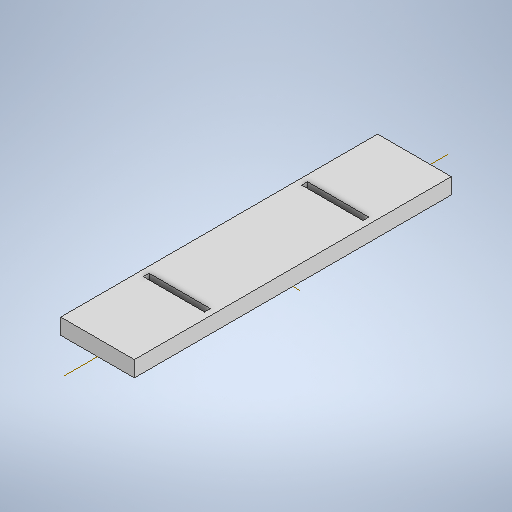
# Autodesk Inventor part: end_wall
Saved by Autodesk Inventor 2025 (Build 290162000, 162)
## iProperties
Created: 2024-04-06
Part Number: end_wall
Material: 일반
Document SubType Name: Modeling
Designer: gmsee
Density: 1 g/cm^3
Appearance: 기본값
Author: gmsee
Autodesk Inventor part; units mm, degrees
ref_plane "YZ Plane" through (0, 0, 0) normal (1, 0, 0) x (0, 1, 0)
ref_plane "XZ Plane" through (0, 0, 0) normal (0, 1, 0) x (-1, 0, 0)
ref_plane "XY Plane" through (0, 0, 0) normal (0, 0, 1) x (1, 0, 0)
sketch "스케치1" plane through (0, 0, 0) normal (0, 1, 0) x (-1, 0, 0)
  line L0 (23.25, 0) -> (23.25, -100)
  line L1 (23.25, -100) -> (0, -100)
  line L2 (32.55, 0) -> (-32.55, 0) projected
  line L3 (0, -144) -> (0, 164) projected
  line L4 (0, -48.15) -> (19.35, -48.15)
  line L5 (19.35, -48.15) -> (19.35, -51.85)
  line L6 (19.35, -51.85) -> (0, -51.85)
  line L7 (23.25, 0) -> (23.25, 100)
  line L8 (23.25, 100) -> (0, 100)
  line L9 (0, 144) -> (0, -164)
  line L10 (0, 48.15) -> (19.35, 48.15)
  line L11 (19.35, 48.15) -> (19.35, 51.85)
  line L12 (19.35, 51.85) -> (0, 51.85)
  line L13 (-23.25, 0) -> (-23.25, -100)
  line L14 (-23.25, -100) -> (0, -100)
  line L15 (-32.55, 0) -> (32.55, 0)
  line L16 (0, -48.15) -> (-19.35, -48.15)
  line L17 (-19.35, -48.15) -> (-19.35, -51.85)
  line L18 (-19.35, -51.85) -> (0, -51.85)
  line L19 (-23.25, 0) -> (-23.25, 100)
  line L20 (-23.25, 100) -> (0, 100)
  line L21 (0, 48.15) -> (-19.35, 48.15)
  line L22 (-19.35, 48.15) -> (-19.35, 51.85)
  line L23 (-19.35, 51.85) -> (0, 51.85)
  point P0 (0, 0)
  point P1 (11.625, -100)
  point P2 (11.625, 100)
  point P3 (-11.625, -100)
  point P4 (-11.625, 100)
  dimension "d0" = 100
  dimension "d1" = 23.25
  dimension "d2" = 3.7
  dimension "d3" = 19.35
  dimension "d4" = 48.15
  constraints: 44 end point, 20 symmetric about line, 8 point on line, 3 perpendicular, 1 horizontal, 1 midpoint, 1 vertical
  measures "d0" distance of L0.start L0.end
  measures "d1" distance of L0.end L1.end
  measures "d2" distance between parallel lines of L6 L4
  measures "d3" distance of L5.end L6.end
  measures "d4" distance from line of point (11.625, -100) L6
extrude "돌출1" add sketch "스케치1" along normal blind 10 contours L0 L1 L3 L6 L5 L4 L2 | L2 L3 L10 L11 L12 L8 L7 | L3 L16 L17 L18 L14 L13 L2 | L2 L19 L20 L3 L23 L22 L21
